Autodesk Inventor part; units mm, degrees
(part 2 of 4)
  line L920 (-9.1525, 3.1357) -> (-9.3195, 2.955)
  line L921 (-9.1525, 3.1357) -> (-8.9855, 2.955)
  line L922 (-9.3195, 2.955) -> (-9.1525, 2.7688)
  line L923 (-8.9855, 2.955) -> (-9.1525, 2.7688)
  line L924 (-9.1525, 2.6703) -> (-8.9855, 2.4896)
  line L925 (-9.1525, 2.6703) -> (-9.3195, 2.4896)
  line L926 (-8.9855, 2.4896) -> (-9.1525, 2.3035)
  line L927 (-9.3195, 2.4896) -> (-9.1525, 2.3035)
  line L928 (-9.6693, 2.1808) -> (-9.8363, 2.0001)
  line L929 (-9.6693, 2.1808) -> (-9.5023, 2.0001)
  line L930 (-9.8363, 2.0001) -> (-9.6693, 1.8139)
  line L931 (-9.5023, 2.0001) -> (-9.6693, 1.8139)
  line L932 (-9.6693, 1.7094) -> (-9.8363, 1.5287)
  line L933 (-9.6693, 1.7094) -> (-9.5023, 1.5287)
  line L934 (-9.8363, 1.5287) -> (-9.6693, 1.3425)
  line L935 (-9.5023, 1.5287) -> (-9.6693, 1.3425)
  line L936 (-9.1525, 2.1808) -> (-8.9855, 2.0001)
  line L937 (-9.1525, 2.1808) -> (-9.3195, 2.0001)
  line L938 (-9.3195, 2.0001) -> (-9.1525, 1.8139)
  line L939 (-8.9855, 2.0001) -> (-9.1525, 1.8139)
  line L940 (-9.1525, 1.7094) -> (-8.9855, 1.5287)
  line L941 (-9.1525, 1.7094) -> (-9.3195, 1.5287)
  line L942 (-8.9855, 1.5287) -> (-9.1525, 1.3425)
  line L943 (-9.3195, 1.5287) -> (-9.1525, 1.3425)
  line L944 (-9.6693, 1.1085) -> (-9.8363, 0.9278)
  line L945 (-9.8363, 0.9278) -> (-9.6693, 0.7417)
  line L946 (-9.6693, 1.1085) -> (-9.5023, 0.9278)
  line L947 (-9.8363, 0.4502) -> (-9.6693, 0.264)
  line L948 (-9.5023, 0.4502) -> (-9.6693, 0.264)
  line L949 (-9.6693, 0.6309) -> (-9.5023, 0.4502)
  line L950 (-9.5023, 0.9278) -> (-9.6693, 0.7417)
  line L951 (-9.6693, 0.6309) -> (-9.8363, 0.4502)
  line L952 (-9.1525, 1.1085) -> (-9.3195, 0.9278)
  line L953 (-9.1525, 1.1085) -> (-8.9855, 0.9278)
  line L954 (-9.3195, 0.9278) -> (-9.1525, 0.7417)
  line L955 (-8.9855, 0.9278) -> (-9.1525, 0.7417)
  line L956 (-9.1525, 0.6309) -> (-8.9855, 0.4502)
  line L957 (-9.1525, 0.6309) -> (-9.3195, 0.4502)
  line L958 (-9.3195, 0.4502) -> (-9.1525, 0.264)
  line L959 (-8.9855, 0.4502) -> (-9.1525, 0.264)
  line L960 (-8.4997, 8.827) -> (-8.6667, 8.6463)
  line L961 (-8.4997, 8.827) -> (-8.3327, 8.6463)
  line L962 (-8.6667, 8.6463) -> (-8.4997, 8.4602)
  line L963 (-8.1499, 8.6463) -> (-7.9829, 8.4602)
  line L964 (-7.8159, 8.6463) -> (-7.9829, 8.4602)
  line L965 (-7.9829, 8.3637) -> (-7.8159, 8.183)
  line L966 (-7.9829, 8.3637) -> (-8.1499, 8.183)
  line L967 (-8.3327, 8.6463) -> (-8.4997, 8.4602)
  line L968 (-8.6667, 9.1056) -> (-8.4997, 8.9195)
  line L969 (-8.3327, 9.1056) -> (-8.4997, 8.9195)
  line L970 (-8.4997, 9.2863) -> (-8.6667, 9.1056)
  line L971 (-8.4997, 9.2863) -> (-8.3327, 9.1056)
  line L972 (-8.6667, 9.5833) -> (-8.4997, 9.3971)
  line L973 (-8.4997, 9.764) -> (-8.3327, 9.5833)
  line L974 (-8.4997, 9.764) -> (-8.6667, 9.5833)
  line L975 (-8.3327, 9.5833) -> (-8.4997, 9.3971)
  line L976 (-7.8159, 7.7177) -> (-7.9829, 7.5315)
  line L977 (-8.6667, 5.8018) -> (-8.4997, 5.6157)
  line L978 (-8.3327, 5.8018) -> (-8.4997, 5.6157)
  line L979 (-8.4997, 5.4909) -> (-8.6667, 5.3102)
  line L980 (-8.4997, 5.4909) -> (-8.3327, 5.3102)
  line L981 (-7.9829, 5.4909) -> (-8.1499, 5.3102)
  line L982 (-8.3327, 5.3102) -> (-8.4997, 5.124)
  line L983 (-7.9829, 5.4909) -> (-7.8159, 5.3102)
  line L984 (-8.1499, 5.3102) -> (-7.9829, 5.124)
  line L985 (-7.8159, 5.3102) -> (-7.9829, 5.124)
  line L986 (-8.6667, 5.3102) -> (-8.4997, 5.124)
  line L987 (-8.4997, 4.5539) -> (-8.6667, 4.3732)
  line L988 (-8.4997, 4.5539) -> (-8.3327, 4.3732)
  line L989 (-8.6667, 4.8325) -> (-8.4997, 4.6463)
  line L990 (-8.4997, 5.0132) -> (-8.3327, 4.8325)
  line L991 (-7.9829, 5.0132) -> (-8.1499, 4.8325)
  line L992 (-7.9829, 5.0132) -> (-7.8159, 4.8325)
  line L993 (-8.4997, 5.0132) -> (-8.6667, 4.8325)
  line L994 (-8.3327, 4.8325) -> (-8.4997, 4.6463)
  line L995 (-7.8159, 4.8325) -> (-7.9829, 4.6463)
  line L996 (-8.1499, 4.8325) -> (-7.9829, 4.6463)
  line L997 (-8.6667, 4.3732) -> (-8.4997, 4.187)
  line L998 (-8.3327, 4.3732) -> (-8.4997, 4.187)
  line L999 (-7.9829, 4.5539) -> (-8.1499, 4.3732)
  line L1000 (-7.9829, 4.5539) -> (-7.8159, 4.3732)
  line L1001 (-8.1499, 4.3732) -> (-7.9829, 4.187)
  line L1002 (-7.8159, 4.3732) -> (-7.9829, 4.187)
  line L1003 (-7.9829, 2.6703) -> (-7.8159, 2.4896)
  line L1004 (-7.9829, 2.6703) -> (-8.1499, 2.4896)
  line L1005 (-8.1499, 2.4896) -> (-7.9829, 2.3035)
  line L1006 (-7.8159, 2.4896) -> (-7.9829, 2.3035)
  line L1007 (-7.9829, 2.1808) -> (-8.1499, 2.0001)
  line L1008 (-7.9829, 2.1808) -> (-7.8159, 2.0001)
  line L1009 (-8.1499, 2.0001) -> (-7.9829, 1.8139)
  line L1010 (-7.8159, 2.0001) -> (-7.9829, 1.8139)
  line L1011 (-7.583, 2.0001) -> (-7.416, 1.8139)
  line L1012 (-7.416, 1.7094) -> (-7.583, 1.5287)
  line L1013 (-7.583, 1.5287) -> (-7.416, 1.3425)
  line L1014 (-7.249, 1.5287) -> (-7.416, 1.3425)
  line L1015 (-7.416, 1.7094) -> (-7.249, 1.5287)
  line L1016 (-7.416, 2.1808) -> (-7.583, 2.0001)
  line L1017 (-7.249, 2.0001) -> (-7.416, 1.8139)
  line L1018 (-7.416, 2.1808) -> (-7.249, 2.0001)
  line L1019 (-7.9829, 0.6309) -> (-8.1499, 0.4502)
  line L1020 (-8.1499, 0.4502) -> (-7.9829, 0.264)
  line L1021 (-8.1499, 0.9278) -> (-7.9829, 0.7417)
  line L1022 (-7.9829, 1.1085) -> (-8.1499, 0.9278)
  line L1023 (-7.9829, 0.6309) -> (-7.8159, 0.4502)
  line L1024 (-7.8159, 0.9278) -> (-7.9829, 0.7417)
  line L1025 (-7.9829, 1.1085) -> (-7.8159, 0.9278)
  line L1026 (-7.416, 0.6309) -> (-7.583, 0.4502)
  line L1027 (-7.583, 0.4502) -> (-7.416, 0.264)
  line L1028 (-7.583, 0.9278) -> (-7.416, 0.7417)
  line L1029 (-7.416, 1.1085) -> (-7.583, 0.9278)
  line L1030 (-7.416, 1.1085) -> (-7.249, 0.9278)
  line L1031 (-7.249, 0.9278) -> (-7.416, 0.7417)
  line L1032 (-7.416, 0.6309) -> (-7.249, 0.4502)
  line L1033 (-7.249, 0.4502) -> (-7.416, 0.264)
  line L1034 (-7.8159, 0.4502) -> (-7.9829, 0.264)
  line L1035 (-7.8159, 8.183) -> (-7.9829, 7.9969)
  line L1036 (-8.1499, 8.183) -> (-7.9829, 7.9969)
  line L1037 (-8.4997, 8.3637) -> (-8.3327, 8.183)
  line L1038 (-8.4997, 8.3637) -> (-8.6667, 8.183)
  line L1039 (-7.9829, 7.8983) -> (-7.8159, 7.7177)
  line L1040 (-8.3327, 8.183) -> (-8.4997, 7.9969)
  line L1041 (-8.6667, 8.183) -> (-8.4997, 7.9969)
  line L1042 (-7.9829, 7.8983) -> (-8.1499, 7.7177)
  line L1043 (-8.4997, 7.8983) -> (-8.3327, 7.7177)
  line L1044 (-8.1499, 7.7177) -> (-7.9829, 7.5315)
  line L1045 (-8.4997, 7.8983) -> (-8.6667, 7.7177)
  line L1046 (-8.6667, 7.7177) -> (-8.4997, 7.5315)
  line L1047 (-8.3327, 7.7177) -> (-8.4997, 7.5315)
  line L1048 (-7.249, 6.7628) -> (-7.416, 6.5766)
  line L1049 (-7.416, 6.9434) -> (-7.249, 6.7628)
  line L1050 (-7.416, 6.4539) -> (-7.583, 6.2732)
  line L1051 (-7.583, 6.2732) -> (-7.416, 6.0871)
  line L1052 (-7.416, 6.4539) -> (-7.249, 6.2732)
  line L1053 (-7.0661, 6.7628) -> (-6.8991, 6.5766)
  line L1054 (-6.8991, 6.9434) -> (-7.0661, 6.7628)
  line L1055 (-6.8991, 6.9434) -> (-6.7321, 6.7628)
  line L1056 (-6.7321, 6.7628) -> (-6.8991, 6.5766)
  line L1057 (-6.8991, 6.4539) -> (-7.0661, 6.2732)
  line L1058 (-6.8991, 6.4539) -> (-6.7321, 6.2732)
  line L1059 (-7.249, 6.2732) -> (-7.416, 6.0871)
  line L1060 (-8.4997, 7.4088) -> (-8.6667, 7.2281)
  line L1061 (-8.6667, 7.2281) -> (-8.4997, 7.042)
  line L1062 (-8.4997, 7.4088) -> (-8.3327, 7.2281)
  line L1063 (-8.3327, 7.2281) -> (-8.4997, 7.042)
  line L1064 (-7.9829, 7.4088) -> (-7.8159, 7.2281)
  line L1065 (-7.9829, 7.4088) -> (-8.1499, 7.2281)
  line L1066 (-8.1499, 7.2281) -> (-7.9829, 7.042)
  line L1067 (-7.8159, 7.2281) -> (-7.9829, 7.042)
  line L1068 (-7.583, 6.7628) -> (-7.416, 6.5766)
  line L1069 (-7.8159, 6.7628) -> (-7.9829, 6.5766)
  line L1070 (-7.9829, 6.9434) -> (-7.8159, 6.7628)
  line L1071 (-8.1499, 6.7628) -> (-7.9829, 6.5766)
  line L1072 (-7.9829, 6.9434) -> (-8.1499, 6.7628)
  line L1073 (-7.416, 6.9434) -> (-7.583, 6.7628)
  line L1074 (-6.8991, 5.9825) -> (-7.0661, 5.8018)
  line L1075 (-7.0661, 5.8018) -> (-6.8991, 5.6157)
  line L1076 (-6.7321, 5.8018) -> (-6.8991, 5.6157)
  line L1077 (-6.8991, 5.9825) -> (-6.7321, 5.8018)
  line L1078 (-8.4997, 6.9434) -> (-8.6667, 6.7628)
  line L1079 (-8.6667, 6.7628) -> (-8.4997, 6.5766)
  line L1080 (-8.4997, 6.9434) -> (-8.3327, 6.7628)
  line L1081 (-8.3327, 6.7628) -> (-8.4997, 6.5766)
  line L1082 (-8.4997, 5.9825) -> (-8.6667, 5.8018)
  line L1083 (-8.4997, 5.9825) -> (-8.3327, 5.8018)
  line L1084 (-8.3327, 6.2732) -> (-8.4997, 6.0871)
  line L1085 (-8.4997, 6.4539) -> (-8.6667, 6.2732)
  line L1086 (-8.4997, 6.4539) -> (-8.3327, 6.2732)
  line L1087 (-8.6667, 6.2732) -> (-8.4997, 6.0871)
  line L1088 (-8.4997, 4.0906) -> (-8.6667, 3.9099)
  line L1089 (-8.4997, 4.0906) -> (-8.3327, 3.9099)
  line L1090 (-8.6667, 3.9099) -> (-8.4997, 3.7237)
  line L1091 (-8.3327, 3.9099) -> (-8.4997, 3.7237)
  line L1092 (-7.9829, 4.0906) -> (-8.1499, 3.9099)
  line L1093 (-7.9829, 4.0906) -> (-7.8159, 3.9099)
  line L1094 (-8.1499, 3.9099) -> (-7.9829, 3.7237)
  line L1095 (-7.8159, 3.9099) -> (-7.9829, 3.7237)
  line L1096 (-7.9829, 3.6252) -> (-8.1499, 3.4445)
  line L1097 (-7.9829, 3.6252) -> (-7.8159, 3.4445)
  line L1098 (-8.1499, 3.4445) -> (-7.9829, 3.2584)
  line L1099 (-7.8159, 3.4445) -> (-7.9829, 3.2584)
  line L1100 (-7.583, 3.4445) -> (-7.416, 3.2584)
  line L1101 (-7.416, 3.6252) -> (-7.583, 3.4445)
  line L1102 (-8.4997, 2.1808) -> (-8.6667, 2.0001)
  line L1103 (-8.4997, 2.1808) -> (-8.3327, 2.0001)
  line L1104 (-8.6667, 2.0001) -> (-8.4997, 1.8139)
  line L1105 (-7.9829, 1.7094) -> (-7.8159, 1.5287)
  line L1106 (-7.8159, 1.5287) -> (-7.9829, 1.3425)
  line L1107 (-7.9829, 1.7094) -> (-8.1499, 1.5287)
  line L1108 (-8.1499, 1.5287) -> (-7.9829, 1.3425)
  line L1109 (-8.4997, 1.7094) -> (-8.3327, 1.5287)
  line L1110 (-8.3327, 1.5287) -> (-8.4997, 1.3425)
  line L1111 (-8.4997, 1.7094) -> (-8.6667, 1.5287)
  line L1112 (-8.6667, 1.5287) -> (-8.4997, 1.3425)
  line L1113 (-8.3327, 2.0001) -> (-8.4997, 1.8139)
  line L1114 (-8.4997, 3.6252) -> (-8.6667, 3.4445)
  line L1115 (-8.4997, 3.6252) -> (-8.3327, 3.4445)
  line L1116 (-8.6667, 3.4445) -> (-8.4997, 3.2584)
  line L1117 (-8.3327, 3.4445) -> (-8.4997, 3.2584)
  line L1118 (-8.4997, 3.1357) -> (-8.6667, 2.955)
  line L1119 (-8.4997, 3.1357) -> (-8.3327, 2.955)
  line L1120 (-8.6667, 2.955) -> (-8.4997, 2.7688)
  line L1121 (-8.3327, 2.4896) -> (-8.4997, 2.3035)
  line L1122 (-8.6667, 2.4896) -> (-8.4997, 2.3035)
  line L1123 (-8.4997, 2.6703) -> (-8.3327, 2.4896)
  line L1124 (-8.4997, 2.6703) -> (-8.6667, 2.4896)
  line L1125 (-8.1499, 2.955) -> (-7.9829, 2.7688)
  line L1126 (-7.8159, 2.955) -> (-7.9829, 2.7688)
  line L1127 (-7.9829, 3.1357) -> (-7.8159, 2.955)
  line L1128 (-7.9829, 3.1357) -> (-8.1499, 2.955)
  line L1129 (-8.3327, 2.955) -> (-8.4997, 2.7688)
  line L1130 (-7.9829, 9.764) -> (-8.1499, 9.5833)
  line L1131 (-8.1499, 9.5833) -> (-7.9829, 9.3971)
  line L1132 (-7.9829, 9.764) -> (-7.8159, 9.5833)
  line L1133 (-7.9829, 8.827) -> (-8.1499, 8.6463)
  line L1134 (-7.9829, 8.827) -> (-7.8159, 8.6463)
  line L1135 (-7.8159, 9.1056) -> (-7.9829, 8.9195)
  line L1136 (-7.9829, 9.2863) -> (-8.1499, 9.1056)
  line L1137 (-7.9829, 9.2863) -> (-7.8159, 9.1056)
  line L1138 (-7.8159, 9.5833) -> (-7.9829, 9.3971)
  line L1139 (-8.1499, 9.1056) -> (-7.9829, 8.9195)
  line L1140 (-7.249, 9.1056) -> (-7.416, 8.9195)
  line L1141 (-7.583, 9.1056) -> (-7.416, 8.9195)
  line L1142 (-6.8991, 9.2863) -> (-7.0661, 9.1056)
  line L1143 (-6.8991, 9.2863) -> (-6.7321, 9.1056)
  line L1144 (-6.7321, 9.1056) -> (-6.8991, 8.9195)
  line L1145 (-7.0661, 9.1056) -> (-6.8991, 8.9195)
  line L1146 (-7.416, 9.2863) -> (-7.249, 9.1056)
  line L1147 (-7.416, 9.2863) -> (-7.583, 9.1056)
  line L1148 (-7.416, 9.764) -> (-7.583, 9.5833)
  line L1149 (-7.583, 9.5833) -> (-7.416, 9.3971)
  line L1150 (-7.249, 9.5833) -> (-7.416, 9.3971)
  line L1151 (-7.416, 9.764) -> (-7.249, 9.5833)
  line L1152 (-7.0661, 9.5833) -> (-6.8991, 9.3971)
  line L1153 (-6.7321, 9.5833) -> (-6.8991, 9.3971)
  line L1154 (-6.8991, 9.764) -> (-7.0661, 9.5833)
  line L1155 (-6.8991, 9.764) -> (-6.7321, 9.5833)
  line L1156 (-6.8991, 5.4909) -> (-7.0661, 5.3102)
  line L1157 (-6.8991, 5.4909) -> (-6.7321, 5.3102)
  line L1158 (-7.0661, 5.3102) -> (-6.8991, 5.124)
  line L1159 (-6.7321, 5.3102) -> (-6.8991, 5.124)
  line L1160 (-7.416, 5.0132) -> (-7.249, 4.8325)
  line L1161 (-7.416, 5.0132) -> (-7.583, 4.8325)
  line L1162 (-7.583, 4.8325) -> (-7.416, 4.6463)
  line L1163 (-7.249, 4.8325) -> (-7.416, 4.6463)
  line L1164 (-6.8991, 5.0132) -> (-7.0661, 4.8325)
  line L1165 (-6.8991, 5.0132) -> (-6.7321, 4.8325)
  line L1166 (-7.0661, 4.8325) -> (-6.8991, 4.6463)
  line L1167 (-6.7321, 4.8325) -> (-6.8991, 4.6463)
  line L1168 (-6.8991, 4.5539) -> (-6.7321, 4.3732)
  line L1169 (-6.8991, 4.5539) -> (-7.0661, 4.3732)
  line L1170 (-7.416, 4.5539) -> (-7.249, 4.3732)
  line L1171 (-7.416, 4.5539) -> (-7.583, 4.3732)
  line L1172 (-6.7321, 4.3732) -> (-6.8991, 4.187)
  line L1173 (-7.583, 4.3732) -> (-7.416, 4.187)
  line L1174 (-7.249, 4.3732) -> (-7.416, 4.187)
  line L1175 (-7.0661, 4.3732) -> (-6.8991, 4.187)
  line L1176 (-6.8991, 4.0906) -> (-6.7321, 3.9099)
  line L1177 (-6.8991, 4.0906) -> (-7.0661, 3.9099)
  line L1178 (-7.416, 4.0906) -> (-7.249, 3.9099)
  line L1179 (-7.416, 4.0906) -> (-7.583, 3.9099)
  line L1180 (-7.416, 8.827) -> (-7.249, 8.6463)
  line L1181 (-7.416, 8.827) -> (-7.583, 8.6463)
  line L1182 (-7.249, 8.6463) -> (-7.416, 8.4602)
  line L1183 (-7.583, 8.6463) -> (-7.416, 8.4602)
  line L1184 (-6.8991, 8.827) -> (-7.0661, 8.6463)
  line L1185 (-6.8991, 8.827) -> (-6.7321, 8.6463)
  line L1186 (-7.0661, 8.6463) -> (-6.8991, 8.4602)
  line L1187 (-6.7321, 8.6463) -> (-6.8991, 8.4602)
  line L1188 (-7.416, 8.3637) -> (-7.249, 8.183)
  line L1189 (-7.416, 8.3637) -> (-7.583, 8.183)
  line L1190 (-7.583, 8.183) -> (-7.416, 7.9969)
  line L1191 (-7.249, 8.183) -> (-7.416, 7.9969)
  line L1192 (-6.8991, 8.3637) -> (-7.0661, 8.183)
  line L1193 (-6.8991, 8.3637) -> (-6.7321, 8.183)
  line L1194 (-7.0661, 8.183) -> (-6.8991, 7.9969)
  line L1195 (-6.7321, 8.183) -> (-6.8991, 7.9969)
  line L1196 (-7.416, 7.8983) -> (-7.583, 7.7177)
  line L1197 (-7.583, 7.7177) -> (-7.416, 7.5315)
  line L1198 (-7.416, 7.8983) -> (-7.249, 7.7177)
  line L1199 (-7.249, 7.7177) -> (-7.416, 7.5315)
  line L1200 (-6.8991, 7.8983) -> (-7.0661, 7.7177)
  line L1201 (-7.0661, 7.7177) -> (-6.8991, 7.5315)
  line L1202 (-6.8991, 7.8983) -> (-6.7321, 7.7177)
  line L1203 (-6.7321, 7.7177) -> (-6.8991, 7.5315)
  line L1204 (-7.416, 7.4088) -> (-7.583, 7.2281)
  line L1205 (-7.583, 7.2281) -> (-7.416, 7.042)
  line L1206 (-6.8991, 7.4088) -> (-7.0661, 7.2281)
  line L1207 (-6.8991, 7.4088) -> (-6.7321, 7.2281)
  line L1208 (-7.416, 7.4088) -> (-7.249, 7.2281)
  line L1209 (-6.7321, 7.2281) -> (-6.8991, 7.042)
  line L1210 (-7.0661, 7.2281) -> (-6.8991, 7.042)
  line L1211 (-7.249, 7.2281) -> (-7.416, 7.042)
  line L1212 (-7.0661, 6.2732) -> (-6.8991, 6.0871)
  line L1213 (-6.7321, 6.2732) -> (-6.8991, 6.0871)
  line L1214 (-7.583, 3.9099) -> (-7.416, 3.7237)
  line L1215 (-7.249, 3.4445) -> (-7.416, 3.2584)
  line L1216 (-7.416, 3.6252) -> (-7.249, 3.4445)
  line L1217 (-7.249, 3.9099) -> (-7.416, 3.7237)
  line L1218 (-7.0661, 3.4445) -> (-6.8991, 3.2584)
  line L1219 (-6.8991, 3.6252) -> (-7.0661, 3.4445)
  line L1220 (-6.8991, 3.1357) -> (-7.0661, 2.955)
  line L1221 (-7.0661, 3.9099) -> (-6.8991, 3.7237)
  line L1222 (-6.7321, 3.9099) -> (-6.8991, 3.7237)
  line L1223 (-6.8991, 3.6252) -> (-6.7321, 3.4445)
  line L1224 (-6.8991, 3.1357) -> (-6.7321, 2.955)
  line L1225 (-6.7321, 3.4445) -> (-6.8991, 3.2584)
  line L1226 (-7.9829, 6.4539) -> (-8.1499, 6.2732)
  line L1227 (-7.9829, 6.4539) -> (-7.8159, 6.2732)
  line L1228 (-8.1499, 6.2732) -> (-7.9829, 6.0871)
  line L1229 (-7.416, 5.9825) -> (-7.249, 5.8018)
  line L1230 (-7.249, 5.8018) -> (-7.416, 5.6157)
  line L1231 (-7.416, 5.9825) -> (-7.583, 5.8018)
  line L1232 (-7.583, 5.8018) -> (-7.416, 5.6157)
  line L1233 (-7.416, 5.4909) -> (-7.249, 5.3102)
  line L1234 (-7.249, 5.3102) -> (-7.416, 5.124)
  line L1235 (-7.583, 5.3102) -> (-7.416, 5.124)
  line L1236 (-7.416, 5.4909) -> (-7.583, 5.3102)
  line L1237 (-7.8159, 6.2732) -> (-7.9829, 6.0871)
  line L1238 (-7.9829, 5.9825) -> (-7.8159, 5.8018)
  line L1239 (-7.8159, 5.8018) -> (-7.9829, 5.6157)
  line L1240 (-7.9829, 5.9825) -> (-8.1499, 5.8018)
  line L1241 (-8.1499, 5.8018) -> (-7.9829, 5.6157)
  line L1242 (-6.8991, 2.1808) -> (-6.7321, 2.0001)
  line L1243 (-6.7321, 2.0001) -> (-6.8991, 1.8139)
  line L1244 (-7.0661, 2.0001) -> (-6.8991, 1.8139)
  line L1245 (-6.8991, 2.1808) -> (-7.0661, 2.0001)
  line L1246 (-7.416, 3.1357) -> (-7.249, 2.955)
  line L1247 (-7.416, 3.1357) -> (-7.583, 2.955)
  line L1248 (-7.0661, 2.955) -> (-6.8991, 2.7688)
  line L1249 (-6.7321, 2.955) -> (-6.8991, 2.7688)
  line L1250 (-7.249, 2.955) -> (-7.416, 2.7688)
  line L1251 (-7.583, 2.955) -> (-7.416, 2.7688)
  line L1252 (-6.8991, 2.6703) -> (-7.0661, 2.4896)
  line L1253 (-6.8991, 2.6703) -> (-6.7321, 2.4896)
  line L1254 (-6.7321, 2.4896) -> (-6.8991, 2.3035)
  line L1255 (-7.0661, 2.4896) -> (-6.8991, 2.3035)
  line L1256 (-7.416, 2.6703) -> (-7.249, 2.4896)
  line L1257 (-7.416, 2.6703) -> (-7.583, 2.4896)
  line L1258 (-7.249, 2.4896) -> (-7.416, 2.3035)
  line L1259 (-7.583, 2.4896) -> (-7.416, 2.3035)
  line L1260 (-6.8991, 1.1085) -> (-7.0661, 0.9278)
  line L1261 (-6.8991, 1.1085) -> (-6.7321, 0.9278)
  line L1262 (-7.0661, 0.9278) -> (-6.8991, 0.7417)
  line L1263 (-6.8991, 0.6309) -> (-7.0661, 0.4502)
  line L1264 (-6.8991, 0.6309) -> (-6.7321, 0.4502)
  line L1265 (-7.0661, 0.4502) -> (-6.8991, 0.264)
  line L1266 (-6.7321, 0.4502) -> (-6.8991, 0.264)
  line L1267 (-6.7321, 0.9278) -> (-6.8991, 0.7417)
  line L1268 (-6.8991, 1.7094) -> (-7.0661, 1.5287)
  line L1269 (-6.7321, 1.5287) -> (-6.8991, 1.3425)
  line L1270 (-6.8991, 1.7094) -> (-6.7321, 1.5287)
  line L1271 (-7.0661, 1.5287) -> (-6.8991, 1.3425)
  line L1272 (-8.4997, 1.1085) -> (-8.6667, 0.9278)
  line L1273 (-8.6667, 0.9278) -> (-8.4997, 0.7417)
  line L1274 (-8.4997, 1.1085) -> (-8.3327, 0.9278)
  line L1275 (-8.6667, 0.4502) -> (-8.4997, 0.264)
  line L1276 (-8.3327, 0.4502) -> (-8.4997, 0.264)
  line L1277 (-8.4997, 0.6309) -> (-8.3327, 0.4502)
  line L1278 (-8.3327, 0.9278) -> (-8.4997, 0.7417)
  line L1279 (-8.4997, 0.6309) -> (-8.6667, 0.4502)
  line L1280 (-6.5651, 9.764) -> (-6.7321, 9.5833)
  line L1281 (-6.7321, 9.5833) -> (-6.5651, 9.3971)
  line L1282 (-6.5651, 9.764) -> (-6.3981, 9.5833)
  line L1283 (-6.3981, 9.5833) -> (-6.5651, 9.3971)
  line L1284 (-6.5651, 9.2863) -> (-6.7321, 9.1056)
  line L1285 (-6.7321, 9.1056) -> (-6.5651, 8.9195)
  line L1286 (-6.5651, 9.2863) -> (-6.3981, 9.1056)
  line L1287 (-6.3981, 9.1056) -> (-6.5651, 8.9195)
  line L1288 (-6.5651, 8.827) -> (-6.7321, 8.6463)
  line L1289 (-6.7321, 8.6463) -> (-6.5651, 8.4602)
  line L1290 (-6.5651, 8.827) -> (-6.3981, 8.6463)
  line L1291 (-6.3981, 8.6463) -> (-6.5651, 8.4602)
  line L1292 (-6.5651, 8.3637) -> (-6.7321, 8.183)
  line L1293 (-6.7321, 8.183) -> (-6.5651, 7.9969)
  line L1294 (-6.5651, 8.3637) -> (-6.3981, 8.183)
  line L1295 (-6.3981, 8.183) -> (-6.5651, 7.9969)
  line L1296 (-6.5651, 7.8983) -> (-6.7321, 7.7177)
  line L1297 (-6.7321, 7.7177) -> (-6.5651, 7.5315)
  line L1298 (-6.5651, 7.8983) -> (-6.3981, 7.7177)
  line L1299 (-6.3981, 7.7177) -> (-6.5651, 7.5315)
  line L1300 (-6.5651, 7.4088) -> (-6.7321, 7.2281)
  line L1301 (-6.7321, 7.2281) -> (-6.5651, 7.042)
  line L1302 (-6.5651, 7.4088) -> (-6.3981, 7.2281)
  line L1303 (-6.3981, 7.2281) -> (-6.5651, 7.042)
  line L1304 (-6.5651, 6.9434) -> (-6.7321, 6.7628)
  line L1305 (-6.7321, 6.7628) -> (-6.5651, 6.5766)
  line L1306 (-6.5651, 6.9434) -> (-6.3981, 6.7628)
  line L1307 (-6.3981, 6.7628) -> (-6.5651, 6.5766)
  line L1308 (-6.5651, 6.4539) -> (-6.7321, 6.2732)
  line L1309 (-6.7321, 6.2732) -> (-6.5651, 6.0871)
  line L1310 (-6.5651, 6.4539) -> (-6.3981, 6.2732)
  line L1311 (-6.3981, 6.2732) -> (-6.5651, 6.0871)
  line L1312 (-6.5651, 5.9825) -> (-6.7321, 5.8018)
  line L1313 (-6.7321, 5.8018) -> (-6.5651, 5.6157)
  line L1314 (-6.5651, 5.9825) -> (-6.3981, 5.8018)
  line L1315 (-6.3981, 5.8018) -> (-6.5651, 5.6157)
  line L1316 (-6.5651, 5.4909) -> (-6.7321, 5.3102)
  line L1317 (-6.7321, 5.3102) -> (-6.5651, 5.124)
  line L1318 (-6.5651, 5.4909) -> (-6.3981, 5.3102)
  line L1319 (-6.5651, 4.5539) -> (-6.7321, 4.3732)
  line L1320 (-6.5651, 4.5539) -> (-6.3981, 4.3732)
  line L1321 (-6.7321, 4.8325) -> (-6.5651, 4.6463)
  line L1322 (-6.3981, 4.8325) -> (-6.5651, 4.6463)
  line L1323 (-6.5651, 5.0132) -> (-6.3981, 4.8325)
  line L1324 (-6.3981, 5.3102) -> (-6.5651, 5.124)
  line L1325 (-6.5651, 5.0132) -> (-6.7321, 4.8325)
  line L1326 (-6.7321, 4.3732) -> (-6.5651, 4.187)
  line L1327 (-6.3981, 4.3732) -> (-6.5651, 4.187)
  line L1328 (-6.5651, 4.0906) -> (-6.7321, 3.9099)
  line L1329 (-6.5651, 4.0906) -> (-6.3981, 3.9099)
  line L1330 (-6.7321, 3.9099) -> (-6.5651, 3.7237)
  line L1331 (-6.3981, 3.9099) -> (-6.5651, 3.7237)
  line L1332 (-6.5651, 3.6252) -> (-6.7321, 3.4445)
  line L1333 (-6.5651, 3.6252) -> (-6.3981, 3.4445)
  line L1334 (-6.7321, 3.4445) -> (-6.5651, 3.2584)
  line L1335 (-6.3981, 3.4445) -> (-6.5651, 3.2584)
  line L1336 (-6.5651, 3.1357) -> (-6.7321, 2.955)
  line L1337 (-6.5651, 3.1357) -> (-6.3981, 2.955)
  line L1338 (-6.7321, 2.955) -> (-6.5651, 2.7688)
  line L1339 (-6.3981, 2.955) -> (-6.5651, 2.7688)
  line L1340 (-6.5651, 2.6703) -> (-6.3981, 2.4896)
  line L1341 (-6.5651, 2.6703) -> (-6.7321, 2.4896)
  line L1342 (-6.3981, 2.4896) -> (-6.5651, 2.3035)
  line L1343 (-6.7321, 2.4896) -> (-6.5651, 2.3035)
  line L1344 (-6.5651, 2.1808) -> (-6.7321, 2.0001)
  line L1345 (-6.5651, 2.1808) -> (-6.3981, 2.0001)
  line L1346 (-6.7321, 2.0001) -> (-6.5651, 1.8139)
  line L1347 (-6.3981, 2.0001) -> (-6.5651, 1.8139)
  line L1348 (-6.5651, 1.7094) -> (-6.7321, 1.5287)
  line L1349 (-6.5651, 1.7094) -> (-6.3981, 1.5287)
  line L1350 (-6.7321, 1.5287) -> (-6.5651, 1.3425)
  line L1351 (-6.3981, 1.5287) -> (-6.5651, 1.3425)
  line L1352 (-6.5651, 1.1085) -> (-6.7321, 0.9278)
  line L1353 (-6.7321, 0.9278) -> (-6.5651, 0.7417)
  line L1354 (-6.5651, 1.1085) -> (-6.3981, 0.9278)
  line L1355 (-6.7321, 0.4502) -> (-6.5651, 0.264)
  line L1356 (-6.3981, 0.4502) -> (-6.5651, 0.264)
  line L1357 (-6.5651, 0.6309) -> (-6.3981, 0.4502)
  line L1358 (-6.3981, 0.9278) -> (-6.5651, 0.7417)
  line L1359 (-6.5651, 0.6309) -> (-6.7321, 0.4502)
  line L1360 (-6.0483, 9.764) -> (-6.2153, 9.5833)
  line L1361 (-6.2153, 9.5833) -> (-6.0483, 9.3971)
  line L1362 (-6.0483, 9.764) -> (-5.8813, 9.5833)
  line L1363 (-6.0483, 8.827) -> (-6.2153, 8.6463)
  line L1364 (-6.0483, 8.827) -> (-5.8813, 8.6463)
  line L1365 (-5.8813, 9.1056) -> (-6.0483, 8.9195)
  line L1366 (-6.0483, 9.2863) -> (-6.2153, 9.1056)
  line L1367 (-6.0483, 9.2863) -> (-5.8813, 9.1056)
  line L1368 (-5.8813, 9.5833) -> (-6.0483, 9.3971)
  line L1369 (-6.2153, 9.1056) -> (-6.0483, 8.9195)
  line L1370 (-6.2153, 8.6463) -> (-6.0483, 8.4602)
  line L1371 (-5.8813, 8.6463) -> (-6.0483, 8.4602)
  line L1372 (-6.0483, 8.3637) -> (-6.2153, 8.183)
  line L1373 (-6.0483, 8.3637) -> (-5.8813, 8.183)
  line L1374 (-6.2153, 8.183) -> (-6.0483, 7.9969)
  line L1375 (-5.8813, 8.183) -> (-6.0483, 7.9969)
  line L1376 (-6.0483, 7.8983) -> (-6.2153, 7.7177)
  line L1377 (-6.2153, 7.7177) -> (-6.0483, 7.5315)
  line L1378 (-5.8813, 7.7177) -> (-6.0483, 7.5315)
  line L1379 (-6.0483, 7.8983) -> (-5.8813, 7.7177)
  line L1380 (-6.0483, 7.4088) -> (-5.8813, 7.2281)
  line L1381 (-6.0483, 7.4088) -> (-6.2153, 7.2281)
  line L1382 (-6.2153, 7.2281) -> (-6.0483, 7.042)
  line L1383 (-5.8813, 7.2281) -> (-6.0483, 7.042)
  line L1384 (-6.0483, 6.9434) -> (-5.8813, 6.7628)
  line L1385 (-5.8813, 6.7628) -> (-6.0483, 6.5766)
  line L1386 (-6.2153, 6.7628) -> (-6.0483, 6.5766)
  line L1387 (-6.0483, 6.9434) -> (-6.2153, 6.7628)
  line L1388 (-6.0483, 6.4539) -> (-6.2153, 6.2732)
  line L1389 (-6.0483, 6.4539) -> (-5.8813, 6.2732)
  line L1390 (-6.2153, 6.2732) -> (-6.0483, 6.0871)
  line L1391 (-5.8813, 6.2732) -> (-6.0483, 6.0871)
  line L1392 (-6.0483, 5.9825) -> (-6.2153, 5.8018)
  line L1393 (-6.0483, 5.9825) -> (-5.8813, 5.8018)
  line L1394 (-6.2153, 5.8018) -> (-6.0483, 5.6157)
  line L1395 (-5.8813, 5.8018) -> (-6.0483, 5.6157)
  line L1396 (-6.0483, 5.4909) -> (-6.2153, 5.3102)
  line L1397 (-6.0483, 5.4909) -> (-5.8813, 5.3102)
  line L1398 (-6.2153, 5.3102) -> (-6.0483, 5.124)
  line L1399 (-5.8813, 5.3102) -> (-6.0483, 5.124)
  line L1400 (-6.0483, 5.0132) -> (-6.2153, 4.8325)
  line L1401 (-6.0483, 5.0132) -> (-5.8813, 4.8325)
  line L1402 (-6.2153, 4.8325) -> (-6.0483, 4.6463)
  line L1403 (-5.8813, 4.8325) -> (-6.0483, 4.6463)
  line L1404 (-6.0483, 4.5539) -> (-5.8813, 4.3732)
  line L1405 (-6.0483, 4.5539) -> (-6.2153, 4.3732)
  line L1406 (-6.2153, 4.3732) -> (-6.0483, 4.187)
  line L1407 (-5.8813, 4.3732) -> (-6.0483, 4.187)
  line L1408 (-6.0483, 4.0906) -> (-6.2153, 3.9099)
  line L1409 (-6.0483, 4.0906) -> (-5.8813, 3.9099)
  line L1410 (-6.2153, 3.9099) -> (-6.0483, 3.7237)
  line L1411 (-5.8813, 3.9099) -> (-6.0483, 3.7237)
  line L1412 (-6.0483, 3.6252) -> (-6.2153, 3.4445)
  line L1413 (-6.0483, 3.6252) -> (-5.8813, 3.4445)
  line L1414 (-6.2153, 3.4445) -> (-6.0483, 3.2584)
  line L1415 (-5.8813, 3.4445) -> (-6.0483, 3.2584)
  line L1416 (-6.0483, 3.1357) -> (-6.2153, 2.955)
  line L1417 (-6.0483, 3.1357) -> (-5.8813, 2.955)
  line L1418 (-6.2153, 2.955) -> (-6.0483, 2.7688)
  line L1419 (-5.8813, 2.955) -> (-6.0483, 2.7688)
  line L1420 (-6.0483, 2.6703) -> (-5.8813, 2.4896)
  line L1421 (-6.0483, 2.6703) -> (-6.2153, 2.4896)
  line L1422 (-6.2153, 2.4896) -> (-6.0483, 2.3035)
  line L1423 (-5.8813, 2.4896) -> (-6.0483, 2.3035)
  line L1424 (-6.0483, 1.1085) -> (-6.2153, 0.9278)
  line L1425 (-6.0483, 1.1085) -> (-5.8813, 0.9278)
  line L1426 (-6.2153, 0.9278) -> (-6.0483, 0.7417)
  line L1427 (-6.0483, 0.6309) -> (-5.8813, 0.4502)
  line L1428 (-6.0483, 0.6309) -> (-6.2153, 0.4502)
  line L1429 (-6.2153, 0.4502) -> (-6.0483, 0.264)
  line L1430 (-5.8813, 0.4502) -> (-6.0483, 0.264)
  line L1431 (-5.8813, 0.9278) -> (-6.0483, 0.7417)
  line L1432 (-6.0483, 2.1808) -> (-5.8813, 2.0001)
  line L1433 (-6.0483, 2.1808) -> (-6.2153, 2.0001)
  line L1434 (-6.2153, 2.0001) -> (-6.0483, 1.8139)
  line L1435 (-5.8813, 2.0001) -> (-6.0483, 1.8139)
  line L1436 (-6.0483, 1.7094) -> (-5.8813, 1.5287)
  line L1437 (-6.0483, 1.7094) -> (-6.2153, 1.5287)
  line L1438 (-5.8813, 1.5287) -> (-6.0483, 1.3425)
  line L1439 (-6.2153, 1.5287) -> (-6.0483, 1.3425)
  line L1440 (-4.9646, 9.2863) -> (-5.1316, 9.1056)
  line L1441 (-4.9646, 9.2863) -> (-4.7976, 9.1056)
  line L1442 (-4.7976, 9.1056) -> (-4.9646, 8.9195)
  line L1443 (-5.1316, 9.1056) -> (-4.9646, 8.9195)
  line L1444 (-4.9646, 8.827) -> (-4.7976, 8.6463)
  line L1445 (-4.9646, 8.827) -> (-5.1316, 8.6463)
  line L1446 (-5.4814, 9.2863) -> (-5.3144, 9.1056)
  line L1447 (-5.4814, 9.2863) -> (-5.6484, 9.1056)
  line L1448 (-5.3144, 9.1056) -> (-5.4814, 8.9195)
  line L1449 (-5.6484, 9.1056) -> (-5.4814, 8.9195)
  line L1450 (-5.4814, 9.764) -> (-5.6484, 9.5833)
  line L1451 (-5.6484, 9.5833) -> (-5.4814, 9.3971)
  line L1452 (-5.3144, 9.5833) -> (-5.4814, 9.3971)
  line L1453 (-5.4814, 9.764) -> (-5.3144, 9.5833)
  line L1454 (-5.1316, 9.5833) -> (-4.9646, 9.3971)
  line L1455 (-4.7976, 9.5833) -> (-4.9646, 9.3971)
  line L1456 (-4.9646, 9.764) -> (-5.1316, 9.5833)
  line L1457 (-4.9646, 9.764) -> (-4.7976, 9.5833)
  line L1458 (-5.4814, 7.4088) -> (-5.6484, 7.2281)
  line L1459 (-5.6484, 7.2281) -> (-5.4814, 7.042)
  line L1460 (-5.4814, 6.4539) -> (-5.3144, 6.2732)
  line L1461 (-5.4814, 6.4539) -> (-5.6484, 6.2732)
  line L1462 (-5.3144, 6.2732) -> (-5.4814, 6.0871)
  line L1463 (-5.6484, 6.2732) -> (-5.4814, 6.0871)
  line L1464 (-4.9646, 5.9825) -> (-4.7976, 5.8018)
  line L1465 (-4.9646, 5.9825) -> (-5.1316, 5.8018)
  line L1466 (-4.7976, 5.8018) -> (-4.9646, 5.6157)
  line L1467 (-5.1316, 5.8018) -> (-4.9646, 5.6157)
  line L1468 (-5.4814, 5.9825) -> (-5.3144, 5.8018)
  line L1469 (-5.4814, 5.9825) -> (-5.6484, 5.8018)
  line L1470 (-5.3144, 5.8018) -> (-5.4814, 5.6157)
  line L1471 (-5.6484, 5.8018) -> (-5.4814, 5.6157)
  line L1472 (-5.1316, 4.8325) -> (-4.9646, 4.6463)
  line L1473 (-4.7976, 4.8325) -> (-4.9646, 4.6463)
  line L1474 (-5.4814, 5.0132) -> (-5.3144, 4.8325)
  line L1475 (-5.4814, 5.0132) -> (-5.6484, 4.8325)
  line L1476 (-4.9646, 4.5539) -> (-4.7976, 4.3732)
  line L1477 (-4.9646, 4.5539) -> (-5.1316, 4.3732)
  line L1478 (-5.3144, 4.8325) -> (-5.4814, 4.6463)
  line L1479 (-5.6484, 4.8325) -> (-5.4814, 4.6463)
  line L1480 (-5.4814, 4.5539) -> (-5.3144, 4.3732)
  line L1481 (-5.4814, 4.5539) -> (-5.6484, 4.3732)
  line L1482 (-5.3144, 3.4445) -> (-5.4814, 3.2584)
  line L1483 (-5.6484, 3.4445) -> (-5.4814, 3.2584)
  line L1484 (-5.4814, 3.6252) -> (-5.3144, 3.4445)
  line L1485 (-5.4814, 3.6252) -> (-5.6484, 3.4445)
  line L1486 (-5.6484, 3.9099) -> (-5.4814, 3.7237)
  line L1487 (-5.4814, 4.0906) -> (-5.3144, 3.9099)
  line L1488 (-5.4814, 4.0906) -> (-5.6484, 3.9099)
  line L1489 (-5.3144, 3.9099) -> (-5.4814, 3.7237)
  line L1490 (-5.4814, 8.827) -> (-5.6484, 8.6463)
  line L1491 (-5.6484, 8.6463) -> (-5.4814, 8.4602)
  line L1492 (-5.4814, 8.827) -> (-5.3144, 8.6463)
  line L1493 (-5.3144, 8.6463) -> (-5.4814, 8.4602)
  line L1494 (-5.4814, 8.3637) -> (-5.6484, 8.183)
  line L1495 (-5.6484, 8.183) -> (-5.4814, 7.9969)
  line L1496 (-5.4814, 8.3637) -> (-5.3144, 8.183)
  line L1497 (-4.7976, 8.6463) -> (-4.9646, 8.4602)
  line L1498 (-5.1316, 8.6463) -> (-4.9646, 8.4602)
  line L1499 (-4.9646, 8.3637) -> (-4.7976, 8.183)
  line L1500 (-4.7976, 8.183) -> (-4.9646, 7.9969)
  line L1501 (-5.1316, 8.183) -> (-4.9646, 7.9969)
  line L1502 (-5.3144, 8.183) -> (-5.4814, 7.9969)
  line L1503 (-4.9646, 8.3637) -> (-5.1316, 8.183)
  line L1504 (-5.4814, 7.8983) -> (-5.6484, 7.7177)
  line L1505 (-5.6484, 7.7177) -> (-5.4814, 7.5315)
  line L1506 (-5.4814, 7.4088) -> (-5.3144, 7.2281)
  line L1507 (-5.3144, 7.2281) -> (-5.4814, 7.042)
  line L1508 (-5.3144, 7.7177) -> (-5.4814, 7.5315)
  line L1509 (-5.4814, 7.8983) -> (-5.3144, 7.7177)
  line L1510 (-4.9646, 6.9434) -> (-5.1316, 6.7628)
  line L1511 (-4.9646, 6.9434) -> (-4.7976, 6.7628)
  line L1512 (-4.9646, 7.4088) -> (-5.1316, 7.2281)
  line L1513 (-4.7976, 7.2281) -> (-4.9646, 7.042)
  line L1514 (-5.1316, 7.7177) -> (-4.9646, 7.5315)
  line L1515 (-4.9646, 7.8983) -> (-5.1316, 7.7177)
  line L1516 (-4.9646, 7.8983) -> (-4.7976, 7.7177)
  line L1517 (-4.7976, 7.7177) -> (-4.9646, 7.5315)
  line L1518 (-4.9646, 7.4088) -> (-4.7976, 7.2281)
  line L1519 (-5.1316, 7.2281) -> (-4.9646, 7.042)
  line L1520 (-5.4814, 6.9434) -> (-5.6484, 6.7628)
  line L1521 (-5.6484, 6.7628) -> (-5.4814, 6.5766)
  line L1522 (-5.4814, 6.9434) -> (-5.3144, 6.7628)
  line L1523 (-5.3144, 6.7628) -> (-5.4814, 6.5766)
  line L1524 (-5.1316, 6.2732) -> (-4.9646, 6.0871)
  line L1525 (-4.7976, 6.2732) -> (-4.9646, 6.0871)
  line L1526 (-4.9646, 6.4539) -> (-5.1316, 6.2732)
  line L1527 (-4.9646, 6.4539) -> (-4.7976, 6.2732)
  line L1528 (-5.1316, 6.7628) -> (-4.9646, 6.5766)
  line L1529 (-4.7976, 6.7628) -> (-4.9646, 6.5766)
  line L1530 (-5.4814, 5.4909) -> (-5.6484, 5.3102)
  line L1531 (-5.6484, 5.3102) -> (-5.4814, 5.124)
  line L1532 (-5.4814, 5.4909) -> (-5.3144, 5.3102)
  line L1533 (-4.9646, 5.0132) -> (-5.1316, 4.8325)
  line L1534 (-5.3144, 5.3102) -> (-5.4814, 5.124)
  line L1535 (-5.1316, 5.3102) -> (-4.9646, 5.124)
  line L1536 (-4.7976, 5.3102) -> (-4.9646, 5.124)
  line L1537 (-4.9646, 5.4909) -> (-5.1316, 5.3102)
  line L1538 (-4.9646, 5.4909) -> (-4.7976, 5.3102)
  line L1539 (-4.9646, 5.0132) -> (-4.7976, 4.8325)
  line L1540 (-5.6484, 4.3732) -> (-5.4814, 4.187)
  line L1541 (-5.3144, 4.3732) -> (-5.4814, 4.187)
  line L1542 (-5.1316, 4.3732) -> (-4.9646, 4.187)
  line L1543 (-4.7976, 4.3732) -> (-4.9646, 4.187)
  line L1544 (-4.9646, 4.0906) -> (-5.1316, 3.9099)
  line L1545 (-4.9646, 4.0906) -> (-4.7976, 3.9099)
  line L1546 (-4.7976, 3.9099) -> (-4.9646, 3.7237)
  line L1547 (-4.9646, 3.6252) -> (-5.1316, 3.4445)
  line L1548 (-4.9646, 3.6252) -> (-4.7976, 3.4445)
  line L1549 (-5.1316, 3.4445) -> (-4.9646, 3.2584)
  line L1550 (-4.7976, 3.4445) -> (-4.9646, 3.2584)
  line L1551 (-5.1316, 3.9099) -> (-4.9646, 3.7237)
  line L1552 (-5.4814, 3.1357) -> (-5.6484, 2.955)
  line L1553 (-5.4814, 3.1357) -> (-5.3144, 2.955)
  line L1554 (-5.6484, 2.955) -> (-5.4814, 2.7688)
  line L1555 (-5.3144, 2.955) -> (-5.4814, 2.7688)
  line L1556 (-5.4814, 2.6703) -> (-5.3144, 2.4896)
  line L1557 (-5.4814, 2.6703) -> (-5.6484, 2.4896)
  line L1558 (-5.3144, 2.4896) -> (-5.4814, 2.3035)
  line L1559 (-5.6484, 2.4896) -> (-5.4814, 2.3035)
  line L1560 (-4.9646, 3.1357) -> (-5.1316, 2.955)
  line L1561 (-4.9646, 3.1357) -> (-4.7976, 2.955)
  line L1562 (-5.1316, 2.955) -> (-4.9646, 2.7688)
  line L1563 (-4.7976, 2.955) -> (-4.9646, 2.7688)
  line L1564 (-4.9646, 2.6703) -> (-4.7976, 2.4896)
  line L1565 (-4.9646, 2.6703) -> (-5.1316, 2.4896)
  line L1566 (-4.7976, 2.4896) -> (-4.9646, 2.3035)
  line L1567 (-5.1316, 2.4896) -> (-4.9646, 2.3035)
  line L1568 (-5.4814, 2.1808) -> (-5.6484, 2.0001)
  line L1569 (-5.4814, 2.1808) -> (-5.3144, 2.0001)
  line L1570 (-5.6484, 2.0001) -> (-5.4814, 1.8139)
  line L1571 (-5.3144, 2.0001) -> (-5.4814, 1.8139)
  line L1572 (-5.4814, 1.7094) -> (-5.6484, 1.5287)
  line L1573 (-5.4814, 1.7094) -> (-5.3144, 1.5287)
  line L1574 (-5.6484, 1.5287) -> (-5.4814, 1.3425)
  line L1575 (-5.3144, 1.5287) -> (-5.4814, 1.3425)
  line L1576 (-4.9646, 2.1808) -> (-4.7976, 2.0001)
  line L1577 (-4.9646, 2.1808) -> (-5.1316, 2.0001)
  line L1578 (-5.1316, 2.0001) -> (-4.9646, 1.8139)
  line L1579 (-4.7976, 2.0001) -> (-4.9646, 1.8139)
  line L1580 (-4.9646, 1.7094) -> (-4.7976, 1.5287)
  line L1581 (-4.9646, 1.7094) -> (-5.1316, 1.5287)
  line L1582 (-4.7976, 1.5287) -> (-4.9646, 1.3425)
  line L1583 (-5.1316, 1.5287) -> (-4.9646, 1.3425)
  line L1584 (-5.4814, 1.1085) -> (-5.6484, 0.9278)
  line L1585 (-5.6484, 0.9278) -> (-5.4814, 0.7417)
  line L1586 (-5.4814, 1.1085) -> (-5.3144, 0.9278)
  line L1587 (-5.6484, 0.4502) -> (-5.4814, 0.264)
  line L1588 (-5.3144, 0.4502) -> (-5.4814, 0.264)
  line L1589 (-5.4814, 0.6309) -> (-5.3144, 0.4502)
  line L1590 (-5.3144, 0.9278) -> (-5.4814, 0.7417)
  line L1591 (-5.4814, 0.6309) -> (-5.6484, 0.4502)
  line L1592 (-4.9646, 1.1085) -> (-5.1316, 0.9278)
  line L1593 (-4.9646, 1.1085) -> (-4.7976, 0.9278)
  line L1594 (-5.1316, 0.9278) -> (-4.9646, 0.7417)
  line L1595 (-4.7976, 0.9278) -> (-4.9646, 0.7417)
  line L1596 (-4.9646, 0.6309) -> (-4.7976, 0.4502)
  line L1597 (-4.9646, 0.6309) -> (-5.1316, 0.4502)
  line L1598 (-5.1316, 0.4502) -> (-4.9646, 0.264)
  line L1599 (-4.7976, 0.4502) -> (-4.9646, 0.264)
  line L1600 (-4.3118, 8.827) -> (-4.4788, 8.6463)
  line L1601 (-4.3118, 8.827) -> (-4.1448, 8.6463)
  line L1602 (-4.4788, 8.6463) -> (-4.3118, 8.4602)
  line L1603 (-3.962, 8.6463) -> (-3.795, 8.4602)
  line L1604 (-3.628, 8.6463) -> (-3.795, 8.4602)
  line L1605 (-3.795, 8.3637) -> (-3.628, 8.183)
  line L1606 (-3.795, 8.3637) -> (-3.962, 8.183)
  line L1607 (-4.1448, 8.6463) -> (-4.3118, 8.4602)
  line L1608 (-4.4788, 9.1056) -> (-4.3118, 8.9195)
  line L1609 (-4.1448, 9.1056) -> (-4.3118, 8.9195)
  line L1610 (-4.3118, 9.2863) -> (-4.4788, 9.1056)
  line L1611 (-4.3118, 9.2863) -> (-4.1448, 9.1056)
  line L1612 (-4.4788, 9.5833) -> (-4.3118, 9.3971)
  line L1613 (-4.3118, 9.764) -> (-4.1448, 9.5833)
  line L1614 (-4.3118, 9.764) -> (-4.4788, 9.5833)
  line L1615 (-4.1448, 9.5833) -> (-4.3118, 9.3971)
  line L1616 (-3.628, 7.7177) -> (-3.795, 7.5315)
  line L1617 (-4.4788, 5.8018) -> (-4.3118, 5.6157)
  line L1618 (-4.1448, 5.8018) -> (-4.3118, 5.6157)
  line L1619 (-4.3118, 5.4909) -> (-4.4788, 5.3102)
  line L1620 (-4.3118, 5.4909) -> (-4.1448, 5.3102)
  line L1621 (-3.795, 5.4909) -> (-3.962, 5.3102)
  line L1622 (-4.1448, 5.3102) -> (-4.3118, 5.124)
  line L1623 (-3.795, 5.4909) -> (-3.628, 5.3102)
  line L1624 (-3.962, 5.3102) -> (-3.795, 5.124)
  line L1625 (-3.628, 5.3102) -> (-3.795, 5.124)
  line L1626 (-4.4788, 5.3102) -> (-4.3118, 5.124)
  line L1627 (-4.3118, 4.5539) -> (-4.4788, 4.3732)
  line L1628 (-4.3118, 4.5539) -> (-4.1448, 4.3732)
  line L1629 (-4.4788, 4.8325) -> (-4.3118, 4.6463)
  line L1630 (-4.3118, 5.0132) -> (-4.1448, 4.8325)
  line L1631 (-3.795, 5.0132) -> (-3.962, 4.8325)
  line L1632 (-3.795, 5.0132) -> (-3.628, 4.8325)
  line L1633 (-4.3118, 5.0132) -> (-4.4788, 4.8325)
  line L1634 (-4.1448, 4.8325) -> (-4.3118, 4.6463)
  line L1635 (-3.628, 4.8325) -> (-3.795, 4.6463)
  line L1636 (-3.962, 4.8325) -> (-3.795, 4.6463)
  line L1637 (-4.4788, 4.3732) -> (-4.3118, 4.187)
  line L1638 (-4.1448, 4.3732) -> (-4.3118, 4.187)
  line L1639 (-3.795, 4.5539) -> (-3.962, 4.3732)
  line L1640 (-3.795, 4.5539) -> (-3.628, 4.3732)
  line L1641 (-3.962, 4.3732) -> (-3.795, 4.187)
  line L1642 (-3.628, 4.3732) -> (-3.795, 4.187)
  line L1643 (-3.795, 2.6703) -> (-3.628, 2.4896)
  line L1644 (-3.795, 2.6703) -> (-3.962, 2.4896)
  line L1645 (-3.962, 2.4896) -> (-3.795, 2.3035)
  line L1646 (-3.628, 2.4896) -> (-3.795, 2.3035)
  line L1647 (-3.795, 2.1808) -> (-3.962, 2.0001)
  line L1648 (-3.795, 2.1808) -> (-3.628, 2.0001)
  line L1649 (-3.962, 2.0001) -> (-3.795, 1.8139)
  line L1650 (-3.628, 2.0001) -> (-3.795, 1.8139)
  line L1651 (-3.3951, 2.0001) -> (-3.2281, 1.8139)
  line L1652 (-3.2281, 1.7094) -> (-3.3951, 1.5287)
  line L1653 (-3.3951, 1.5287) -> (-3.2281, 1.3425)
  line L1654 (-3.0611, 1.5287) -> (-3.2281, 1.3425)
  line L1655 (-3.2281, 1.7094) -> (-3.0611, 1.5287)
  line L1656 (-3.2281, 2.1808) -> (-3.3951, 2.0001)
  line L1657 (-3.0611, 2.0001) -> (-3.2281, 1.8139)
  line L1658 (-3.2281, 2.1808) -> (-3.0611, 2.0001)
  line L1659 (-3.795, 0.6309) -> (-3.962, 0.4502)
  line L1660 (-3.962, 0.4502) -> (-3.795, 0.264)
  line L1661 (-3.962, 0.9278) -> (-3.795, 0.7417)
  line L1662 (-3.795, 1.1085) -> (-3.962, 0.9278)
  line L1663 (-3.795, 0.6309) -> (-3.628, 0.4502)
  line L1664 (-3.628, 0.9278) -> (-3.795, 0.7417)
  line L1665 (-3.795, 1.1085) -> (-3.628, 0.9278)
  line L1666 (-3.2281, 0.6309) -> (-3.3951, 0.4502)
  line L1667 (-3.3951, 0.4502) -> (-3.2281, 0.264)
  line L1668 (-3.3951, 0.9278) -> (-3.2281, 0.7417)
  line L1669 (-3.2281, 1.1085) -> (-3.3951, 0.9278)
  line L1670 (-3.2281, 1.1085) -> (-3.0611, 0.9278)
  line L1671 (-3.0611, 0.9278) -> (-3.2281, 0.7417)
  line L1672 (-3.2281, 0.6309) -> (-3.0611, 0.4502)
  line L1673 (-3.0611, 0.4502) -> (-3.2281, 0.264)
  line L1674 (-3.628, 0.4502) -> (-3.795, 0.264)
  line L1675 (-3.628, 8.183) -> (-3.795, 7.9969)
  line L1676 (-3.962, 8.183) -> (-3.795, 7.9969)
  line L1677 (-4.3118, 8.3637) -> (-4.1448, 8.183)
  line L1678 (-4.3118, 8.3637) -> (-4.4788, 8.183)
  line L1679 (-3.795, 7.8983) -> (-3.628, 7.7177)
  line L1680 (-4.1448, 8.183) -> (-4.3118, 7.9969)
  line L1681 (-4.4788, 8.183) -> (-4.3118, 7.9969)
  line L1682 (-3.795, 7.8983) -> (-3.962, 7.7177)
  line L1683 (-4.3118, 7.8983) -> (-4.1448, 7.7177)
  line L1684 (-3.962, 7.7177) -> (-3.795, 7.5315)
  line L1685 (-4.3118, 7.8983) -> (-4.4788, 7.7177)
  line L1686 (-4.4788, 7.7177) -> (-4.3118, 7.5315)
  line L1687 (-4.1448, 7.7177) -> (-4.3118, 7.5315)
  line L1688 (-3.0611, 6.7628) -> (-3.2281, 6.5766)
  line L1689 (-3.2281, 6.9434) -> (-3.0611, 6.7628)
  line L1690 (-3.2281, 6.4539) -> (-3.3951, 6.2732)
  line L1691 (-3.3951, 6.2732) -> (-3.2281, 6.0871)
  line L1692 (-3.2281, 6.4539) -> (-3.0611, 6.2732)
  line L1693 (-2.8783, 6.7628) -> (-2.7113, 6.5766)
  line L1694 (-2.7113, 6.9434) -> (-2.8783, 6.7628)
  line L1695 (-2.7113, 6.9434) -> (-2.5443, 6.7628)
  line L1696 (-2.5443, 6.7628) -> (-2.7113, 6.5766)
  line L1697 (-2.7113, 6.4539) -> (-2.8783, 6.2732)
  line L1698 (-2.7113, 6.4539) -> (-2.5443, 6.2732)
  line L1699 (-3.0611, 6.2732) -> (-3.2281, 6.0871)
  line L1700 (-4.3118, 7.4088) -> (-4.4788, 7.2281)
  line L1701 (-4.4788, 7.2281) -> (-4.3118, 7.042)
  line L1702 (-4.3118, 7.4088) -> (-4.1448, 7.2281)
  line L1703 (-4.1448, 7.2281) -> (-4.3118, 7.042)
  line L1704 (-3.795, 7.4088) -> (-3.628, 7.2281)
  line L1705 (-3.795, 7.4088) -> (-3.962, 7.2281)
  line L1706 (-3.962, 7.2281) -> (-3.795, 7.042)
  line L1707 (-3.628, 7.2281) -> (-3.795, 7.042)
  line L1708 (-3.3951, 6.7628) -> (-3.2281, 6.5766)
  line L1709 (-3.628, 6.7628) -> (-3.795, 6.5766)
  line L1710 (-3.795, 6.9434) -> (-3.628, 6.7628)
  line L1711 (-3.962, 6.7628) -> (-3.795, 6.5766)
  line L1712 (-3.795, 6.9434) -> (-3.962, 6.7628)
  line L1713 (-3.2281, 6.9434) -> (-3.3951, 6.7628)
  line L1714 (-2.7113, 5.9825) -> (-2.8783, 5.8018)
  line L1715 (-2.8783, 5.8018) -> (-2.7113, 5.6157)
  line L1716 (-2.5443, 5.8018) -> (-2.7113, 5.6157)
  line L1717 (-2.7113, 5.9825) -> (-2.5443, 5.8018)
  line L1718 (-4.3118, 6.9434) -> (-4.4788, 6.7628)
  line L1719 (-4.4788, 6.7628) -> (-4.3118, 6.5766)
  line L1720 (-4.3118, 6.9434) -> (-4.1448, 6.7628)
  line L1721 (-4.1448, 6.7628) -> (-4.3118, 6.5766)
  line L1722 (-4.3118, 5.9825) -> (-4.4788, 5.8018)
  line L1723 (-4.3118, 5.9825) -> (-4.1448, 5.8018)
  line L1724 (-4.1448, 6.2732) -> (-4.3118, 6.0871)
  line L1725 (-4.3118, 6.4539) -> (-4.4788, 6.2732)
  line L1726 (-4.3118, 6.4539) -> (-4.1448, 6.2732)
  line L1727 (-4.4788, 6.2732) -> (-4.3118, 6.0871)
  line L1728 (-4.3118, 4.0906) -> (-4.4788, 3.9099)
  line L1729 (-4.3118, 4.0906) -> (-4.1448, 3.9099)
  line L1730 (-4.4788, 3.9099) -> (-4.3118, 3.7237)
  line L1731 (-4.1448, 3.9099) -> (-4.3118, 3.7237)
  line L1732 (-3.795, 4.0906) -> (-3.962, 3.9099)
  line L1733 (-3.795, 4.0906) -> (-3.628, 3.9099)
  line L1734 (-3.962, 3.9099) -> (-3.795, 3.7237)
  line L1735 (-3.628, 3.9099) -> (-3.795, 3.7237)
  line L1736 (-3.795, 3.6252) -> (-3.962, 3.4445)
  line L1737 (-3.795, 3.6252) -> (-3.628, 3.4445)
  line L1738 (-3.962, 3.4445) -> (-3.795, 3.2584)
  line L1739 (-3.628, 3.4445) -> (-3.795, 3.2584)
  line L1740 (-3.3951, 3.4445) -> (-3.2281, 3.2584)
  line L1741 (-3.2281, 3.6252) -> (-3.3951, 3.4445)
  line L1742 (-4.3118, 2.1808) -> (-4.4788, 2.0001)
  line L1743 (-4.3118, 2.1808) -> (-4.1448, 2.0001)
  line L1744 (-4.4788, 2.0001) -> (-4.3118, 1.8139)
  line L1745 (-3.795, 1.7094) -> (-3.628, 1.5287)
  line L1746 (-3.628, 1.5287) -> (-3.795, 1.3425)
  line L1747 (-3.795, 1.7094) -> (-3.962, 1.5287)
  line L1748 (-3.962, 1.5287) -> (-3.795, 1.3425)
  line L1749 (-4.3118, 1.7094) -> (-4.1448, 1.5287)
  line L1750 (-4.1448, 1.5287) -> (-4.3118, 1.3425)
  line L1751 (-4.3118, 1.7094) -> (-4.4788, 1.5287)
  line L1752 (-4.4788, 1.5287) -> (-4.3118, 1.3425)
  line L1753 (-4.1448, 2.0001) -> (-4.3118, 1.8139)
  line L1754 (-4.3118, 3.6252) -> (-4.4788, 3.4445)
  line L1755 (-4.3118, 3.6252) -> (-4.1448, 3.4445)
  line L1756 (-4.4788, 3.4445) -> (-4.3118, 3.2584)
  line L1757 (-4.1448, 3.4445) -> (-4.3118, 3.2584)
  line L1758 (-4.3118, 3.1357) -> (-4.4788, 2.955)
  line L1759 (-4.3118, 3.1357) -> (-4.1448, 2.955)
  line L1760 (-4.4788, 2.955) -> (-4.3118, 2.7688)
  line L1761 (-4.1448, 2.4896) -> (-4.3118, 2.3035)
  line L1762 (-4.4788, 2.4896) -> (-4.3118, 2.3035)
  line L1763 (-4.3118, 2.6703) -> (-4.1448, 2.4896)
  line L1764 (-4.3118, 2.6703) -> (-4.4788, 2.4896)
  line L1765 (-3.962, 2.955) -> (-3.795, 2.7688)
  line L1766 (-3.628, 2.955) -> (-3.795, 2.7688)
  line L1767 (-3.795, 3.1357) -> (-3.628, 2.955)
  line L1768 (-3.795, 3.1357) -> (-3.962, 2.955)
  line L1769 (-4.1448, 2.955) -> (-4.3118, 2.7688)
  line L1770 (-3.795, 9.764) -> (-3.962, 9.5833)
  line L1771 (-3.962, 9.5833) -> (-3.795, 9.3971)
  line L1772 (-3.795, 9.764) -> (-3.628, 9.5833)
  line L1773 (-3.795, 8.827) -> (-3.962, 8.6463)
  line L1774 (-3.795, 8.827) -> (-3.628, 8.6463)
  line L1775 (-3.628, 9.1056) -> (-3.795, 8.9195)
  line L1776 (-3.795, 9.2863) -> (-3.962, 9.1056)
  line L1777 (-3.795, 9.2863) -> (-3.628, 9.1056)
  line L1778 (-3.628, 9.5833) -> (-3.795, 9.3971)
  line L1779 (-3.962, 9.1056) -> (-3.795, 8.9195)
  line L1780 (-3.0611, 9.1056) -> (-3.2281, 8.9195)
  line L1781 (-3.3951, 9.1056) -> (-3.2281, 8.9195)
  line L1782 (-2.7113, 9.2863) -> (-2.8783, 9.1056)
  line L1783 (-2.7113, 9.2863) -> (-2.5443, 9.1056)
  line L1784 (-2.5443, 9.1056) -> (-2.7113, 8.9195)
  line L1785 (-2.8783, 9.1056) -> (-2.7113, 8.9195)
  line L1786 (-3.2281, 9.2863) -> (-3.0611, 9.1056)
  line L1787 (-3.2281, 9.2863) -> (-3.3951, 9.1056)
  line L1788 (-3.2281, 9.764) -> (-3.3951, 9.5833)
  line L1789 (-3.3951, 9.5833) -> (-3.2281, 9.3971)
  line L1790 (-3.0611, 9.5833) -> (-3.2281, 9.3971)
  line L1791 (-3.2281, 9.764) -> (-3.0611, 9.5833)
  line L1792 (-2.8783, 9.5833) -> (-2.7113, 9.3971)
  line L1793 (-2.5443, 9.5833) -> (-2.7113, 9.3971)
  line L1794 (-2.7113, 9.764) -> (-2.8783, 9.5833)
  line L1795 (-2.7113, 9.764) -> (-2.5443, 9.5833)
  line L1796 (-2.7113, 5.4909) -> (-2.8783, 5.3102)
  line L1797 (-2.7113, 5.4909) -> (-2.5443, 5.3102)
  line L1798 (-2.8783, 5.3102) -> (-2.7113, 5.124)
  line L1799 (-2.5443, 5.3102) -> (-2.7113, 5.124)
  line L1800 (-3.2281, 5.0132) -> (-3.0611, 4.8325)
  line L1801 (-3.2281, 5.0132) -> (-3.3951, 4.8325)
  line L1802 (-3.3951, 4.8325) -> (-3.2281, 4.6463)
  line L1803 (-3.0611, 4.8325) -> (-3.2281, 4.6463)
  line L1804 (-2.7113, 5.0132) -> (-2.8783, 4.8325)
  line L1805 (-2.7113, 5.0132) -> (-2.5443, 4.8325)
  line L1806 (-2.8783, 4.8325) -> (-2.7113, 4.6463)
  line L1807 (-2.5443, 4.8325) -> (-2.7113, 4.6463)
  line L1808 (-2.7113, 4.5539) -> (-2.5443, 4.3732)
  line L1809 (-2.7113, 4.5539) -> (-2.8783, 4.3732)
  line L1810 (-3.2281, 4.5539) -> (-3.0611, 4.3732)
  line L1811 (-3.2281, 4.5539) -> (-3.3951, 4.3732)
  line L1812 (-2.5443, 4.3732) -> (-2.7113, 4.187)
  line L1813 (-3.3951, 4.3732) -> (-3.2281, 4.187)
  line L1814 (-3.0611, 4.3732) -> (-3.2281, 4.187)
  line L1815 (-2.8783, 4.3732) -> (-2.7113, 4.187)
  line L1816 (-2.7113, 4.0906) -> (-2.5443, 3.9099)
  line L1817 (-2.7113, 4.0906) -> (-2.8783, 3.9099)
  line L1818 (-3.2281, 4.0906) -> (-3.0611, 3.9099)
  line L1819 (-3.2281, 4.0906) -> (-3.3951, 3.9099)
  line L1820 (-3.2281, 8.827) -> (-3.0611, 8.6463)
  line L1821 (-3.2281, 8.827) -> (-3.3951, 8.6463)
  line L1822 (-3.0611, 8.6463) -> (-3.2281, 8.4602)
  line L1823 (-3.3951, 8.6463) -> (-3.2281, 8.4602)
  line L1824 (-2.7113, 8.827) -> (-2.8783, 8.6463)
  line L1825 (-2.7113, 8.827) -> (-2.5443, 8.6463)
  line L1826 (-2.8783, 8.6463) -> (-2.7113, 8.4602)
  line L1827 (-2.5443, 8.6463) -> (-2.7113, 8.4602)
  line L1828 (-3.2281, 8.3637) -> (-3.0611, 8.183)
  line L1829 (-3.2281, 8.3637) -> (-3.3951, 8.183)
  line L1830 (-3.3951, 8.183) -> (-3.2281, 7.9969)
  line L1831 (-3.0611, 8.183) -> (-3.2281, 7.9969)
  line L1832 (-2.7113, 8.3637) -> (-2.8783, 8.183)
  line L1833 (-2.7113, 8.3637) -> (-2.5443, 8.183)
  line L1834 (-2.8783, 8.183) -> (-2.7113, 7.9969)
  line L1835 (-2.5443, 8.183) -> (-2.7113, 7.9969)
  line L1836 (-3.2281, 7.8983) -> (-3.3951, 7.7177)
  line L1837 (-3.3951, 7.7177) -> (-3.2281, 7.5315)
  line L1838 (-3.2281, 7.8983) -> (-3.0611, 7.7177)
  line L1839 (-3.0611, 7.7177) -> (-3.2281, 7.5315)
  line L1840 (-2.7113, 7.8983) -> (-2.8783, 7.7177)
  line L1841 (-2.8783, 7.7177) -> (-2.7113, 7.5315)
  line L1842 (-2.7113, 7.8983) -> (-2.5443, 7.7177)
  line L1843 (-2.5443, 7.7177) -> (-2.7113, 7.5315)
  line L1844 (-3.2281, 7.4088) -> (-3.3951, 7.2281)
  line L1845 (-3.3951, 7.2281) -> (-3.2281, 7.042)
  line L1846 (-2.7113, 7.4088) -> (-2.8783, 7.2281)
  line L1847 (-2.7113, 7.4088) -> (-2.5443, 7.2281)
  line L1848 (-3.2281, 7.4088) -> (-3.0611, 7.2281)
  line L1849 (-2.5443, 7.2281) -> (-2.7113, 7.042)
  line L1850 (-2.8783, 7.2281) -> (-2.7113, 7.042)
  line L1851 (-3.0611, 7.2281) -> (-3.2281, 7.042)
  line L1852 (-2.8783, 6.2732) -> (-2.7113, 6.0871)
  line L1853 (-2.5443, 6.2732) -> (-2.7113, 6.0871)
  line L1854 (-3.3951, 3.9099) -> (-3.2281, 3.7237)
  line L1855 (-3.0611, 3.4445) -> (-3.2281, 3.2584)
  line L1856 (-3.2281, 3.6252) -> (-3.0611, 3.4445)
  line L1857 (-3.0611, 3.9099) -> (-3.2281, 3.7237)
  line L1858 (-2.8783, 3.4445) -> (-2.7113, 3.2584)
  line L1859 (-2.7113, 3.6252) -> (-2.8783, 3.4445)
  line L1860 (-2.7113, 3.1357) -> (-2.8783, 2.955)
  line L1861 (-2.8783, 3.9099) -> (-2.7113, 3.7237)
  line L1862 (-2.5443, 3.9099) -> (-2.7113, 3.7237)
  line L1863 (-2.7113, 3.6252) -> (-2.5443, 3.4445)
  line L1864 (-2.7113, 3.1357) -> (-2.5443, 2.955)
  line L1865 (-2.5443, 3.4445) -> (-2.7113, 3.2584)
  line L1866 (-3.795, 6.4539) -> (-3.962, 6.2732)
  line L1867 (-3.795, 6.4539) -> (-3.628, 6.2732)
  line L1868 (-3.962, 6.2732) -> (-3.795, 6.0871)
  line L1869 (-3.2281, 5.9825) -> (-3.0611, 5.8018)
  line L1870 (-3.0611, 5.8018) -> (-3.2281, 5.6157)
  line L1871 (-3.2281, 5.9825) -> (-3.3951, 5.8018)
  line L1872 (-3.3951, 5.8018) -> (-3.2281, 5.6157)
  line L1873 (-3.2281, 5.4909) -> (-3.0611, 5.3102)
  line L1874 (-3.0611, 5.3102) -> (-3.2281, 5.124)
  line L1875 (-3.3951, 5.3102) -> (-3.2281, 5.124)
  line L1876 (-3.2281, 5.4909) -> (-3.3951, 5.3102)
  line L1877 (-3.628, 6.2732) -> (-3.795, 6.0871)
  line L1878 (-3.795, 5.9825) -> (-3.628, 5.8018)
  line L1879 (-3.628, 5.8018) -> (-3.795, 5.6157)
  line L1880 (-3.795, 5.9825) -> (-3.962, 5.8018)
  line L1881 (-3.962, 5.8018) -> (-3.795, 5.6157)
  line L1882 (-2.7113, 2.1808) -> (-2.5443, 2.0001)
  line L1883 (-2.5443, 2.0001) -> (-2.7113, 1.8139)
  line L1884 (-2.8783, 2.0001) -> (-2.7113, 1.8139)
  line L1885 (-2.7113, 2.1808) -> (-2.8783, 2.0001)
  line L1886 (-3.2281, 3.1357) -> (-3.0611, 2.955)
  line L1887 (-3.2281, 3.1357) -> (-3.3951, 2.955)
  line L1888 (-2.8783, 2.955) -> (-2.7113, 2.7688)
  line L1889 (-2.5443, 2.955) -> (-2.7113, 2.7688)
  line L1890 (-3.0611, 2.955) -> (-3.2281, 2.7688)
  line L1891 (-3.3951, 2.955) -> (-3.2281, 2.7688)